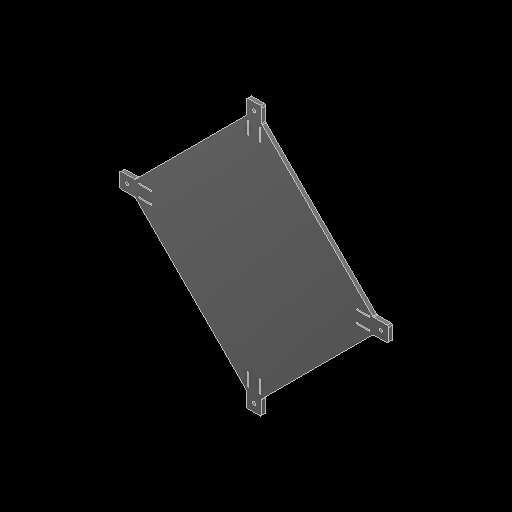
# Autodesk Inventor part: base_plate
Saved by Autodesk Inventor 2026.1 (Build 301233000, 233)
## iProperties
Created: 2025-09-14
Part Number: base_plate
Material: Aluminum 6061
Document SubType Name: Modeling
Designer: drago
Density: 2.7 g/cm^3
Appearance: Smooth - Black
Author: drago
Autodesk Inventor part; units mm, degrees
ref_plane "YZ Plane" through (0, 0, 0) normal (1, 0, 0) x (0, 1, 0)
ref_plane "XZ Plane" through (0, 0, 0) normal (0, 1, 0) x (-1, 0, 0)
ref_plane "XY Plane" through (0, 0, 0) normal (0, 0, 1) x (1, 0, 0)
sketch "Sketch2" plane through (0, 0, 0) normal (0, 0, 1) x (1, 0, 0)
  line L0 (307.5, 20) -> (347.5, 20)
  line L1 (347.5, 20) -> (347.5, -20)
  line L2 (347.5, -20) -> (307.5, -20)
  line L3 (307.5, -20) -> (307.5, 20)
  line L4 (307.5, 20) -> (347.5, -20) construction
  line L5 (347.5, 20) -> (307.5, -20) construction
  line L6 (327.5, 0) -> (-327.5, 0) construction
  line L7 (0, -327.5) -> (0, 327.5) construction
  line L8 (327.5, 0) -> (327.5, 0) construction
  line L9 (327.5, 4.25) -> (327.5, 4.25)
  line L10 (327.5, -4.25) -> (327.5, -4.25)
  arc A0 (327.5, -4.25) -> (327.5, 4.25) centre (327.5, 0) ccw
  arc A1 (327.5, 4.25) -> (327.5, -4.25) centre (327.5, 0) ccw
  line L11 (266.2, 15.5) -> (297.2, 15.5) construction
  line L12 (266.2, 13.9) -> (297.2, 13.9)
  line L13 (297.2, 17.1) -> (266.2, 17.1)
  arc A2 (266.2, 17.1) -> (266.2, 13.9) centre (266.2, 15.5) ccw
  arc A3 (297.2, 13.9) -> (297.2, 17.1) centre (297.2, 15.5) ccw
  line L14 (266.2, -15.5) -> (297.2, -15.5) construction
  line L15 (266.2, -17.1) -> (297.2, -17.1)
  line L16 (297.2, -13.9) -> (266.2, -13.9)
  arc A4 (266.2, -13.9) -> (266.2, -17.1) centre (266.2, -15.5) ccw
  arc A5 (297.2, -17.1) -> (297.2, -13.9) centre (297.2, -15.5) ccw
  arc A6 (-4.25, 327.5) -> (4.25, 327.5) centre (0, 327.5) ccw
  line L17 (-13.9, 266.2) -> (-13.9, 297.2)
  line L18 (-15.5, 266.2) -> (-15.5, 297.2) construction
  line L19 (-17.1, 297.2) -> (-17.1, 266.2)
  line L20 (17.1, 266.2) -> (17.1, 297.2)
  line L21 (13.9, 297.2) -> (13.9, 266.2)
  arc A7 (17.1, 297.2) -> (13.9, 297.2) centre (15.5, 297.2) ccw
  line L22 (20, 307.5) -> (-20, 307.5)
  line L23 (15.5, 266.2) -> (15.5, 297.2) construction
  arc A8 (-17.1, 266.2) -> (-13.9, 266.2) centre (-15.5, 266.2) ccw
  arc A9 (13.9, 266.2) -> (17.1, 266.2) centre (15.5, 266.2) ccw
  line L24 (-20, 307.5) -> (-20, 347.5)
  line L25 (-20, 347.5) -> (20, 347.5)
  line L26 (20, 347.5) -> (20, 307.5)
  line L27 (-20, 307.5) -> (20, 347.5) construction
  line L28 (-20, 347.5) -> (20, 307.5) construction
  arc A10 (-13.9, 297.2) -> (-17.1, 297.2) centre (-15.5, 297.2) ccw
  line L29 (0, 327.5) -> (0, 327.5) construction
  line L30 (4.25, 327.5) -> (4.25, 327.5)
  arc A11 (4.25, 327.5) -> (-4.25, 327.5) centre (0, 327.5) ccw
  line L31 (-4.25, 327.5) -> (-4.25, 327.5)
  arc A12 (-327.5, -4.25) -> (-327.5, 4.25) centre (-327.5, 0) ccw
  line L32 (-266.2, -13.9) -> (-297.2, -13.9)
  line L33 (-266.2, -15.5) -> (-297.2, -15.5) construction
  line L34 (-297.2, -17.1) -> (-266.2, -17.1)
  line L35 (-266.2, 17.1) -> (-297.2, 17.1)
  line L36 (-297.2, 13.9) -> (-266.2, 13.9)
  arc A13 (-297.2, 17.1) -> (-297.2, 13.9) centre (-297.2, 15.5) ccw
  line L37 (-307.5, 20) -> (-307.5, -20)
  line L38 (-266.2, 15.5) -> (-297.2, 15.5) construction
  arc A14 (-266.2, -17.1) -> (-266.2, -13.9) centre (-266.2, -15.5) ccw
  arc A15 (-266.2, 13.9) -> (-266.2, 17.1) centre (-266.2, 15.5) ccw
  line L39 (-307.5, -20) -> (-347.5, -20)
  line L40 (-347.5, -20) -> (-347.5, 20)
  line L41 (-347.5, 20) -> (-307.5, 20)
  line L42 (-307.5, -20) -> (-347.5, 20) construction
  line L43 (-347.5, -20) -> (-307.5, 20) construction
  arc A16 (-297.2, -13.9) -> (-297.2, -17.1) centre (-297.2, -15.5) ccw
  line L44 (-327.5, 0) -> (-327.5, 0) construction
  line L45 (-327.5, 4.25) -> (-327.5, 4.25)
  arc A17 (-327.5, 4.25) -> (-327.5, -4.25) centre (-327.5, 0) ccw
  line L46 (-327.5, -4.25) -> (-327.5, -4.25)
  arc A18 (4.25, -327.5) -> (-4.25, -327.5) centre (0, -327.5) ccw
  line L47 (13.9, -266.2) -> (13.9, -297.2)
  line L48 (15.5, -266.2) -> (15.5, -297.2) construction
  line L49 (17.1, -297.2) -> (17.1, -266.2)
  line L50 (-17.1, -266.2) -> (-17.1, -297.2)
  line L51 (-13.9, -297.2) -> (-13.9, -266.2)
  arc A19 (-17.1, -297.2) -> (-13.9, -297.2) centre (-15.5, -297.2) ccw
  line L52 (-20, -307.5) -> (20, -307.5)
  line L53 (-15.5, -266.2) -> (-15.5, -297.2) construction
  arc A20 (17.1, -266.2) -> (13.9, -266.2) centre (15.5, -266.2) ccw
  arc A21 (-13.9, -266.2) -> (-17.1, -266.2) centre (-15.5, -266.2) ccw
  line L54 (20, -307.5) -> (20, -347.5)
  line L55 (20, -347.5) -> (-20, -347.5)
  line L56 (-20, -347.5) -> (-20, -307.5)
  line L57 (20, -307.5) -> (-20, -347.5) construction
  line L58 (20, -347.5) -> (-20, -307.5) construction
  arc A22 (13.9, -297.2) -> (17.1, -297.2) centre (15.5, -297.2) ccw
  line L59 (0, -327.5) -> (0, -327.5) construction
  line L60 (-4.25, -327.5) -> (-4.25, -327.5)
  arc A23 (-4.25, -327.5) -> (4.25, -327.5) centre (0, -327.5) ccw
  line L61 (4.25, -327.5) -> (4.25, -327.5)
  line L62 (-307.5, 20) -> (-20, 307.5)
  line L63 (20, 307.5) -> (307.5, 20)
  line L64 (307.5, -20) -> (20, -307.5)
  line L65 (-20, -307.5) -> (-307.5, -20)
  point P0 (0, 0)
  point P1 (327.5, 0)
  point P2 (281.7, 15.5)
  point P3 (281.7, -15.5)
  point P4 (15.5, 281.7)
  point P5 (-15.5, 281.7)
  point P6 (0, 327.5)
  point P7 (-281.7, 15.5)
  point P8 (-281.7, -15.5)
  point P9 (-327.5, 0)
  point P10 (-15.5, -281.7)
  point P11 (15.5, -281.7)
  point P12 (0, -327.5)
  dimension "d148" = 40
  dimension "d149" = 655
  dimension "d154" = 0
  dimension "d155" = 8.5
  dimension "d156" = 31
  dimension "d157" = 3.2
  dimension "d171" = 31
  dimension "d172" = 10.3
  dimension "d173" = 10.3
  dimension "d176" = 360
  constraints: 156 end point, 48 point on circle, 24 centre point, 12 tangent, 7 midpoint, 5 parallel, 4 horizontal, 3 equal length, 3 perpendicular, 2 collinear, 1 equal radius, 1 point on line, 1 vertical, 187 other
  measures "d148" distance of L0.end L1.end
  measures "d149" distance of L6.start L6.end
  measures "d154" distance of L6.start L8.end
  measures "d155" diameter of A1
  measures "d156" distance of L11.start L11.end
  measures "d157" diameter of A3
  measures "d171" distance between parallel lines of L14 L11
  measures "d172" distance from line of L3 L11.end
  measures "d173" distance from line of L3 L14.end
extrude "Extrusion10" add sketch "Sketch2" against normal blind 10
fillet "Fillet8" radius 4 16 edges at (20, 347.5, -5) (-20, 347.5, -5) (-20, 307.5, -5) (-307.5, 20, -5) (-347.5, 20, -5) (-347.5, -20, -5) (347.5, 20, -5) (-20, -307.5, -5) (-20, -347.5, -5) (20, 307.5, -5) (20, -347.5, -5) (347.5, -20, -5) (307.5, -20, -5) (20, -307.5, -5) (307.5, 20, -5) (-307.5, -20, -5)
equation "\"ring_inner_diam\" = 565"
equation "\"ring_outer_diam\" = 615"
equation "\"dist_motor_bar\" = 10.3"
equation "\"motor_slot_diam\" = 3.2"
equation "\"motor_slot_length\" = 31"
equation "\"bar_slot_diam\" = 8.5"
equation "\"bar_slot_length\" = 0"
equation "\"diag_dist_bar_holes_old_fridge\" = 536.791"
equation "\"motor_dist_slots\" = 31"
body "Solid4"
